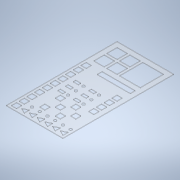
# Autodesk Inventor part: Plexi
Saved by Autodesk Inventor 2021 (Build 250183000, 183)
## iProperties
Created: 2020-07-15
Part Number: Plexi
Material: Generic
Document SubType Name: Modeling
Designer: adick
Density: 1 g/cm^3
Appearance: Default
Author: adick
Autodesk Inventor part; units mm, degrees
ref_plane "YZ Plane" through (0, 0, 0) normal (1, 0, 0) x (0, 1, 0)
ref_plane "XZ Plane" through (0, 0, 0) normal (0, 1, 0) x (-1, 0, 0)
ref_plane "XY Plane" through (0, 0, 0) normal (0, 0, 1) x (1, 0, 0)
sketch "Sketch1" plane through (0, 0, 0) normal (0, 1, 0) x (-1, 0, 0)
  line L0 (0, 0) -> (-220, 0)
  line L1 (-220, 0) -> (-220, -430)
  line L2 (-220, -430) -> (0, -430)
  line L3 (0, -430) -> (0, 0)
  line L4 (0, 0) -> (-10, 0)
  line L5 (0, -10) -> (0, 0)
  line L6 (-40, 0) -> (-30, 0)
  line L7 (-10, -10) -> (-30, -10)
  line L8 (-30, -10) -> (-30, -30)
  line L9 (-30, -30) -> (-10, -30)
  line L10 (-10, -30) -> (-10, -10)
  line L11 (-60, -10) -> (-60, -30)
  line L12 (-90, -10) -> (-90, -30)
  line L13 (-120, -10) -> (-120, -30)
  line L14 (-150, -10) -> (-150, -30)
  line L15 (-180, -10) -> (-180, -30)
  line L16 (-210, -10) -> (-210, -30)
  line L17 (-10, -40) -> (-30, -40)
  line L18 (-30, -40) -> (-30, -60)
  line L19 (-30, -60) -> (-10, -60)
  line L20 (-10, -60) -> (-10, -40)
  line L21 (-30, -70) -> (-10, -70)
  line L22 (-10, -70) -> (-10, -90)
  line L23 (-10, -90) -> (-30, -90)
  line L24 (-30, -90) -> (-30, -70)
  line L25 (-10, -100) -> (-30, -100)
  line L26 (-30, -100) -> (-30, -120)
  line L27 (-30, -120) -> (-10, -120)
  line L28 (-10, -120) -> (-10, -100)
  line L29 (-10, -130) -> (-30, -130)
  line L30 (-30, -130) -> (-30, -150)
  line L31 (-30, -150) -> (-10, -150)
  line L32 (-10, -150) -> (-10, -130)
  line L33 (-30, -160) -> (-10, -160)
  line L34 (-10, -160) -> (-10, -180)
  line L35 (-10, -180) -> (-30, -180)
  line L36 (-30, -180) -> (-30, -160)
  line L37 (-10, -190) -> (-30, -190)
  line L38 (-30, -190) -> (-30, -210)
  line L39 (-30, -210) -> (-10, -210)
  line L40 (-10, -210) -> (-10, -190)
  line L41 (-10, -220) -> (-30, -220)
  line L42 (-30, -220) -> (-30, -240)
  line L43 (-30, -240) -> (-10, -240)
  line L44 (-10, -240) -> (-10, -220)
  line L45 (-10, -250) -> (-30, -250)
  line L46 (-30, -250) -> (-30, -270)
  line L47 (-30, -270) -> (-10, -270)
  line L48 (-10, -270) -> (-10, -250)
  line L49 (-30, -280) -> (-10, -280)
  line L50 (-10, -280) -> (-10, -300)
  line L51 (-10, -300) -> (-30, -300)
  line L52 (-30, -300) -> (-30, -280)
  line L53 (-20, -410) -> (-60, -410)
  line L54 (-60, -410) -> (-60, -370)
  line L55 (-60, -370) -> (-20, -370)
  line L56 (-20, -370) -> (-20, -410)
  line L57 (-20, -360) -> (-60, -360)
  line L58 (-60, -360) -> (-60, -320)
  line L59 (-60, -320) -> (-20, -320)
  line L60 (-20, -320) -> (-20, -360)
  line L61 (-180, -320) -> (-120, -320)
  line L62 (-120, -320) -> (-120, -410)
  line L63 (-70, -320) -> (-110, -320)
  line L64 (-110, -320) -> (-110, -360)
  line L65 (-110, -360) -> (-70, -360)
  line L66 (-70, -360) -> (-70, -320)
  line L67 (-110, -370) -> (-70, -370)
  line L68 (-70, -370) -> (-70, -410)
  line L69 (-70, -410) -> (-110, -410)
  line L70 (-110, -410) -> (-110, -370)
  line L71 (-120, -320) -> (-200, -320)
  line L72 (-200, -320) -> (-200, -410)
  line L73 (-200, -410) -> (-120, -410)
  line L74 (-120, -410) -> (-120, -320)
  line L75 (-40, -20) -> (-60, -30)
  line L76 (-40, -20) -> (-60, -10)
  line L77 (-70, -20) -> (-90, -10)
  line L78 (-70, -20) -> (-90, -30)
  line L79 (-100, -20) -> (-120, -10)
  line L80 (-120, -30) -> (-100, -20)
  line L81 (-130, -20) -> (-150, -10)
  line L82 (-150, -30) -> (-130, -20)
  line L83 (-160, -20) -> (-180, -30)
  line L84 (-160, -20) -> (-180, -10)
  line L85 (-190, -20) -> (-210, -10)
  line L86 (-190, -20) -> (-210, -30)
  line L87 (-200, -300) -> (-72, -300)
  line L88 (-72, -300) -> (-72, -281)
  line L89 (-72, -281) -> (-200, -281)
  line L90 (-200, -281) -> (-200, -300)
  line L91 (-150, -60) -> (-130, -60)
  line L92 (-130, -60) -> (-130, -80)
  line L93 (-130, -80) -> (-150, -80)
  line L94 (-150, -80) -> (-150, -60)
  line L95 (-120, -90) -> (-100, -90)
  line L96 (-100, -90) -> (-100, -110)
  line L97 (-100, -110) -> (-120, -110)
  line L98 (-120, -110) -> (-120, -90)
  line L99 (-130, -120) -> (-150, -120)
  line L100 (-150, -120) -> (-150, -140)
  line L101 (-150, -140) -> (-130, -140)
  line L102 (-130, -140) -> (-130, -120)
  line L103 (-160, -110) -> (-180, -110)
  line L104 (-180, -110) -> (-180, -90)
  line L105 (-180, -90) -> (-160, -90)
  line L106 (-160, -90) -> (-160, -110)
  line L107 (-90, -80) -> (-70, -80)
  line L108 (-70, -80) -> (-70, -60)
  line L109 (-70, -60) -> (-90, -60)
  line L110 (-90, -60) -> (-90, -80)
  line L111 (-90, -120) -> (-70, -120)
  line L112 (-70, -120) -> (-70, -140)
  line L113 (-70, -140) -> (-90, -140)
  line L114 (-90, -140) -> (-90, -120)
  line L115 (-180, -140) -> (-200, -140)
  line L116 (-200, -140) -> (-200, -160)
  line L117 (-200, -160) -> (-180, -160)
  line L118 (-180, -160) -> (-180, -140)
  line L119 (-180, -170) -> (-200, -170)
  line L120 (-200, -170) -> (-200, -190)
  line L121 (-200, -190) -> (-180, -190)
  line L122 (-180, -190) -> (-180, -170)
  line L123 (-180, -200) -> (-200, -200)
  line L124 (-200, -200) -> (-200, -220)
  line L125 (-200, -220) -> (-180, -220)
  line L126 (-180, -220) -> (-180, -200)
  line L127 (-180, -230) -> (-200, -230)
  line L128 (-200, -230) -> (-200, -250)
  line L129 (-200, -250) -> (-180, -250)
  line L130 (-180, -250) -> (-180, -230)
  line L131 (-130, -160) -> (-110, -160)
  line L132 (-110, -160) -> (-110, -150)
  line L133 (-110, -150) -> (-130, -150)
  line L134 (-130, -150) -> (-130, -160)
  line L135 (-130, -190) -> (-110, -190)
  line L136 (-110, -190) -> (-110, -180)
  line L137 (-110, -180) -> (-130, -180)
  line L138 (-130, -180) -> (-130, -190)
  line L139 (-130, -220) -> (-110, -220)
  line L140 (-110, -220) -> (-110, -210)
  line L141 (-110, -210) -> (-130, -210)
  line L142 (-130, -210) -> (-130, -220)
  line L143 (-70, -160) -> (-50, -160)
  line L144 (-50, -160) -> (-50, -150)
  line L145 (-50, -150) -> (-70, -150)
  line L146 (-70, -150) -> (-70, -160)
  line L147 (-70, -190) -> (-50, -190)
  line L148 (-50, -190) -> (-50, -180)
  line L149 (-50, -180) -> (-70, -180)
  line L150 (-70, -180) -> (-70, -190)
  line L151 (-70, -220) -> (-50, -220)
  line L152 (-50, -220) -> (-50, -210)
  line L153 (-50, -210) -> (-70, -210)
  line L154 (-70, -210) -> (-70, -220)
  circle A0 centre (-55, -45) radius 5
  circle A1 centre (-85, -45) radius 5
  circle A2 centre (-115, -45) radius 5
  circle A3 centre (-145, -45) radius 5
  circle A4 centre (-175, -45) radius 5
  circle A5 centre (-205, -45) radius 5
  circle A6 centre (-145, -155) radius 5
  circle A7 centre (-145, -185) radius 5
  circle A8 centre (-145, -215) radius 5
  circle A9 centre (-85, -215) radius 5
  circle A10 centre (-85, -185) radius 5
  circle A11 centre (-85, -155) radius 5
  dimension "d0" = 220
  dimension "d1" = 430
  dimension "d28" = 128
  constraints: 310 end point, 74 parallel, 41 point on line, 34 horizontal, 33 perpendicular, 12 centre point, 1 coincident
  measures "d0" distance of L2.end L1.end
  measures "d1" distance of L1.end L0.end
  measures "d28" distance of L89.end L88.end
extrude "Extrusion1" add sketch "Sketch1" along normal blind 2.5
body "Solid1"
